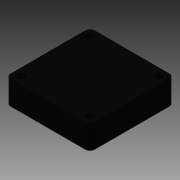
# Autodesk Inventor part: stepper_middle_28
Saved by Autodesk Inventor 2013 (Build 170138000, 138)
## iProperties
Shininess: 20.0
Created: 2013-02-12
Part Number: stepper_middle_28
Document SubType Name: Modeling
Designer: Noa Izumi
Material: Default
Density: 1 g/cm^3
Density: 0.0
Volumn: 0.0
Area: 0.0
PropertySet Name: Model Information
Control State: 0
Master: False
Checked Out: False
Author: Noa Izumi
Autodesk Inventor part; units mm, degrees
ref_plane "YZ Plane" through (0, 0, 0) normal (1, 0, 0) x (0, 1, 0)
ref_plane "XZ Plane" through (0, 0, 0) normal (0, 1, 0) x (-1, 0, 0)
ref_plane "XY Plane" through (0, 0, 0) normal (0, 0, 1) x (1, 0, 0)
sketch "Sketch1" plane through (0, 0, 0) normal (0, 0, 1) x (1, 0, 0)
  line L0 (0, 0) -> (28, 0)
  line L1 (28, 0) -> (28, 28)
  line L2 (28, 28) -> (0, 28)
  line L3 (0, 28) -> (0, 0)
  dimension "d0" = 28
  dimension "d1" = 28
  constraints: 8 end point, 2 parallel, 1 horizontal, 1 perpendicular
  measures "d0" distance of L2.end L0.start
  measures "d1" distance of L0.start L0.end
extrude "Extrusion1" add sketch "Sketch1" along normal blind 8
fillet "Fillet1" radius 1.5 4 edges at (0, 0, 4) (28, 0, 4) (0, 28, 4) (28, 28, 4)
sketch "Sketch3" plane through (0, 0, 8) normal (0, 0, 1) x (1, 0, 0)
  line L0 (1.5, 28) -> (26.5, 28) projected
  line L1 (0, 1.5) -> (0, 26.5) projected
  line L2 (26.5, 0) -> (1.5, 0) projected
  line L3 (28, 26.5) -> (28, 1.5) projected
  point P0 (2.5, 2.5)
  point P1 (25.5, 2.5)
  point P2 (2.5, 25.5)
  point P3 (25.5, 25.5)
  dimension "d10" = 2.5
  dimension "d11" = 2.5
  dimension "d12" = 2.5
  dimension "d13" = 2.5
  dimension "d14" = 2.5
  dimension "d15" = 2.5
  dimension "d16" = 2.5
  dimension "d17" = 2.5
  measures "d10" distance from line of L1 point (2.5, 2.5)
  measures "d11" distance from line of point (2.5, 2.5) L2
  measures "d12" distance from line of point (25.5, 2.5) L2
  measures "d13" distance from line of L3 point (25.5, 2.5)
  measures "d14" distance from line of L1 point (2.5, 25.5)
  measures "d15" distance from line of L0 point (2.5, 25.5)
  measures "d16" distance from line of L0 point (25.5, 25.5)
  measures "d17" distance from line of L3 point (25.5, 25.5)
hole "Hole1" at (2.5, 2.5, 8) at (25.5, 2.5, 8) at (2.5, 25.5, 8) at (25.5, 25.5, 8) direction (0, 0, -1) diameter 2.5 end through all
